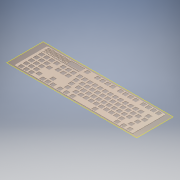
# Autodesk Inventor part: Plate
Saved by Autodesk Inventor 2016 (Build 200138000, 138)
## iProperties
Created: 2021-02-01
Part Number: Plate
Material: Aluminum 6061
Document SubType Name: Modeling
Designer: Tom
Density: 2.7 g/cm^3
Appearance: Aluminum - Flat
Author: Tom
Autodesk Inventor part; units mm, degrees
(part 1 of 4)
ref_plane "YZ Plane" through (0, 0, 0) normal (1, 0, 0) x (0, 1, 0)
ref_plane "XZ Plane" through (0, 0, 0) normal (0, 1, 0) x (-1, 0, 0)
ref_plane "XY Plane" through (0, 0, 0) normal (0, 0, 1) x (1, 0, 0)
ref_plane "Work Plane1" through (-107.46, -92.5006, 10.9251) normal (0, 0, 1) x (1, 0, 0)
sketch "Sketch1" plane through (-107.46, -92.5006, 10.9251) normal (0, 0, 1) x (1, 0, 0)
  line L0 (216.125, 61.75) -> (-216.125, 61.75)
  arc A0 (-216.125, 61.75) -> (-220.875, 57) centre (-216.125, 57) ccw
  line L1 (-220.875, 57) -> (-220.875, -57)
  arc A1 (-220.875, -57) -> (-216.125, -61.75) centre (-216.125, -57) ccw
  line L2 (-216.125, -61.75) -> (216.125, -61.75)
  arc A2 (216.125, -61.75) -> (220.875, -57) centre (216.125, -57) ccw
  line L3 (220.875, -57) -> (220.875, 57)
  arc A3 (220.875, 57) -> (216.125, 61.75) centre (216.125, 57) ccw
  circle A4 centre (216.125, 57) radius 1.35
  circle A5 centre (216.125, 0) radius 1.35
  circle A6 centre (216.125, -57) radius 1.35
  circle A7 centre (118.75, -57) radius 1.35
  circle A8 centre (23.75, -57) radius 1.35
  circle A9 centre (-133.753, -57) radius 1.35
  circle A10 centre (-47.5, -57) radius 1.35
  circle A11 centre (-216.125, -57) radius 1.35
  circle A12 centre (-216.125, 57) radius 1.35
  circle A13 centre (-216.125, 0) radius 1.35
  circle A14 centre (-66.5, -19) radius 1.35
  circle A15 centre (-45.125, 11.875) radius 1.35
  circle A16 centre (-73.625, 57) radius 1.35
  circle A17 centre (-9.5, -24.356) radius 1.35
  circle A18 centre (47.5, 57) radius 1.35
  circle A19 centre (-114, 14.25) radius 1.35
  circle A20 centre (-175.75, 14.25) radius 1.35
  circle A21 centre (-175.75, -23.75) radius 1.35
  circle A22 centre (33.25, 13.49) radius 1.35
  circle A23 centre (76, -23.086) radius 1.35
  circle A24 centre (109.25, 13.49) radius 1.35
  circle A25 centre (166.25, -40.375) radius 1.35
  circle A26 centre (187.625, 11.875) radius 1.35
  circle A27 centre (133, 57) radius 1.35
  line L4 (-78.04, 59.315) -> (-128.84, 59.315)
  line L5 (-128.84, 41.535) -> (-78.04, 41.535)
  line L6 (-78.04, 56.315) -> (-78.04, 44.535)
  line L7 (-78.04, 56.315) -> (-78.04, 59.315)
  line L8 (-78.04, 41.535) -> (-78.04, 44.535)
  line L9 (-128.84, 44.535) -> (-128.84, 41.535)
  line L10 (-128.84, 59.315) -> (-128.84, 56.315)
  line L11 (-128.84, 56.315) -> (-128.84, 44.535)
  line L12 (-78.04, 59.315) -> (-77.34, 59.315)
  line L13 (-77.34, 59.315) -> (-77.34, 41.535)
  line L14 (-77.34, 41.535) -> (-78.04, 41.535)
  line L15 (-128.84, 59.315) -> (-129.54, 59.315)
  line L16 (-129.54, 59.315) -> (-129.54, 41.535)
  line L17 (-129.54, 41.535) -> (-128.84, 41.535)
  line L18 (-62.2, 51.5) -> (-62.2, 50.35)
  line L19 (-62.2, 50.35) -> (-61.3, 50.35)
  line L20 (-61.3, 50.35) -> (-61.3, 51.5)
  arc A28 (-61.1, 51.7) -> (-61.3, 51.5) centre (-61.1, 51.5) ccw
  line L21 (-61.1, 51.7) -> (-59.85, 51.7)
  line L22 (-59.85, 51.7) -> (-59.85, 52.8)
  line L23 (-59.85, 52.8) -> (-61.1, 52.8)
  arc A29 (-61.3, 53) -> (-61.1, 52.8) centre (-61.1, 53) ccw
  line L24 (-61.3, 53) -> (-61.3, 54.15)
  line L25 (-61.3, 54.15) -> (-62.2, 54.15)
  line L26 (-62.2, 54.15) -> (-62.2, 53)
  arc A30 (-62.4, 52.8) -> (-62.2, 53) centre (-62.4, 53) ccw
  line L27 (-62.4, 52.8) -> (-63.65, 52.8)
  line L28 (-63.65, 52.8) -> (-63.65, 51.7)
  line L29 (-63.65, 51.7) -> (-62.4, 51.7)
  arc A31 (-62.2, 51.5) -> (-62.4, 51.7) centre (-62.4, 51.5) ccw
  line L30 (-24.2, 51.5) -> (-24.2, 50.35)
  line L31 (-24.2, 50.35) -> (-23.3, 50.35)
  line L32 (-23.3, 50.35) -> (-23.3, 51.5)
  arc A32 (-23.1, 51.7) -> (-23.3, 51.5) centre (-23.1, 51.5) ccw
  line L33 (-23.1, 51.7) -> (-21.85, 51.7)
  line L34 (-21.85, 51.7) -> (-21.85, 52.8)
  line L35 (-21.85, 52.8) -> (-23.1, 52.8)
  arc A33 (-23.3, 53) -> (-23.1, 52.8) centre (-23.1, 53) ccw
  line L36 (-23.3, 53) -> (-23.3, 54.15)
  line L37 (-23.3, 54.15) -> (-24.2, 54.15)
  line L38 (-24.2, 54.15) -> (-24.2, 53)
  arc A34 (-24.4, 52.8) -> (-24.2, 53) centre (-24.4, 53) ccw
  line L39 (-24.4, 52.8) -> (-25.65, 52.8)
  line L40 (-25.65, 52.8) -> (-25.65, 51.7)
  line L41 (-25.65, 51.7) -> (-24.4, 51.7)
  arc A35 (-24.2, 51.5) -> (-24.4, 51.7) centre (-24.4, 51.5) ccw
  line L42 (-24.2, 23) -> (-24.2, 21.85)
  line L43 (-24.2, 21.85) -> (-23.3, 21.85)
  line L44 (-23.3, 21.85) -> (-23.3, 23)
  arc A36 (-23.1, 23.2) -> (-23.3, 23) centre (-23.1, 23) ccw
  line L45 (-23.1, 23.2) -> (-21.85, 23.2)
  line L46 (-21.85, 23.2) -> (-21.85, 24.3)
  line L47 (-21.85, 24.3) -> (-23.1, 24.3)
  arc A37 (-23.3, 24.5) -> (-23.1, 24.3) centre (-23.1, 24.5) ccw
  line L48 (-23.3, 24.5) -> (-23.3, 25.65)
  line L49 (-23.3, 25.65) -> (-24.2, 25.65)
  line L50 (-24.2, 25.65) -> (-24.2, 24.5)
  arc A38 (-24.4, 24.3) -> (-24.2, 24.5) centre (-24.4, 24.5) ccw
  line L51 (-24.4, 24.3) -> (-25.65, 24.3)
  line L52 (-25.65, 24.3) -> (-25.65, 23.2)
  line L53 (-25.65, 23.2) -> (-24.4, 23.2)
  arc A39 (-24.2, 23) -> (-24.4, 23.2) centre (-24.4, 23) ccw
  line L54 (-43.2, 23) -> (-43.2, 21.85)
  line L55 (-43.2, 21.85) -> (-42.3, 21.85)
  line L56 (-42.3, 21.85) -> (-42.3, 23)
  arc A40 (-42.1, 23.2) -> (-42.3, 23) centre (-42.1, 23) ccw
  line L57 (-42.1, 23.2) -> (-40.85, 23.2)
  line L58 (-40.85, 23.2) -> (-40.85, 24.3)
  line L59 (-40.85, 24.3) -> (-42.1, 24.3)
  arc A41 (-42.3, 24.5) -> (-42.1, 24.3) centre (-42.1, 24.5) ccw
  line L60 (-42.3, 24.5) -> (-42.3, 25.65)
  line L61 (-42.3, 25.65) -> (-43.2, 25.65)
  line L62 (-43.2, 25.65) -> (-43.2, 24.5)
  arc A42 (-43.4, 24.3) -> (-43.2, 24.5) centre (-43.4, 24.5) ccw
  line L63 (-43.4, 24.3) -> (-44.65, 24.3)
  line L64 (-44.65, 24.3) -> (-44.65, 23.2)
  line L65 (-44.65, 23.2) -> (-43.4, 23.2)
  arc A43 (-43.2, 23) -> (-43.4, 23.2) centre (-43.4, 23) ccw
  line L66 (-62.2, 23) -> (-62.2, 21.85)
  line L67 (-62.2, 21.85) -> (-61.3, 21.85)
  line L68 (-61.3, 21.85) -> (-61.3, 23)
  arc A44 (-61.1, 23.2) -> (-61.3, 23) centre (-61.1, 23) ccw
  line L69 (-61.1, 23.2) -> (-59.85, 23.2)
  line L70 (-59.85, 23.2) -> (-59.85, 24.3)
  line L71 (-59.85, 24.3) -> (-61.1, 24.3)
  arc A45 (-61.3, 24.5) -> (-61.1, 24.3) centre (-61.1, 24.5) ccw
  line L72 (-61.3, 24.5) -> (-61.3, 25.65)
  line L73 (-61.3, 25.65) -> (-62.2, 25.65)
  line L74 (-62.2, 25.65) -> (-62.2, 24.5)
  arc A46 (-62.4, 24.3) -> (-62.2, 24.5) centre (-62.4, 24.5) ccw
  line L75 (-62.4, 24.3) -> (-63.65, 24.3)
  line L76 (-63.65, 24.3) -> (-63.65, 23.2)
  line L77 (-63.65, 23.2) -> (-62.4, 23.2)
  arc A47 (-62.2, 23) -> (-62.4, 23.2) centre (-62.4, 23) ccw
  line L78 (-123.95, 23) -> (-123.95, 21.85)
  line L79 (-123.95, 21.85) -> (-123.05, 21.85)
  line L80 (-123.05, 21.85) -> (-123.05, 23)
  arc A48 (-122.85, 23.2) -> (-123.05, 23) centre (-122.85, 23) ccw
  line L81 (-122.85, 23.2) -> (-121.6, 23.2)
  line L82 (-121.6, 23.2) -> (-121.6, 24.3)
  line L83 (-121.6, 24.3) -> (-122.85, 24.3)
  arc A49 (-123.05, 24.5) -> (-122.85, 24.3) centre (-122.85, 24.5) ccw
  line L84 (-123.05, 24.5) -> (-123.05, 25.65)
  line L85 (-123.05, 25.65) -> (-123.95, 25.65)
  line L86 (-123.95, 25.65) -> (-123.95, 24.5)
  arc A50 (-124.15, 24.3) -> (-123.95, 24.5) centre (-124.15, 24.5) ccw
  line L87 (-124.15, 24.3) -> (-125.4, 24.3)
  line L88 (-125.4, 24.3) -> (-125.4, 23.2)
  line L89 (-125.4, 23.2) -> (-124.15, 23.2)
  arc A51 (-123.95, 23) -> (-124.15, 23.2) centre (-124.15, 23) ccw
  line L90 (-104.95, 23) -> (-104.95, 21.85)
  line L91 (-104.95, 21.85) -> (-104.05, 21.85)
  line L92 (-104.05, 21.85) -> (-104.05, 23)
  arc A52 (-103.85, 23.2) -> (-104.05, 23) centre (-103.85, 23) ccw
  line L93 (-103.85, 23.2) -> (-102.6, 23.2)
  line L94 (-102.6, 23.2) -> (-102.6, 24.3)
  line L95 (-102.6, 24.3) -> (-103.85, 24.3)
  arc A53 (-104.05, 24.5) -> (-103.85, 24.3) centre (-103.85, 24.5) ccw
  line L96 (-104.05, 24.5) -> (-104.05, 25.65)
  line L97 (-104.05, 25.65) -> (-104.95, 25.65)
  line L98 (-104.95, 25.65) -> (-104.95, 24.5)
  arc A54 (-105.15, 24.3) -> (-104.95, 24.5) centre (-105.15, 24.5) ccw
  line L99 (-105.15, 24.3) -> (-106.4, 24.3)
  line L100 (-106.4, 24.3) -> (-106.4, 23.2)
  line L101 (-106.4, 23.2) -> (-105.15, 23.2)
  arc A55 (-104.95, 23) -> (-105.15, 23.2) centre (-105.15, 23) ccw
  line L102 (-85.95, 23) -> (-85.95, 21.85)
  line L103 (-85.95, 21.85) -> (-85.05, 21.85)
  line L104 (-85.05, 21.85) -> (-85.05, 23)
  arc A56 (-84.85, 23.2) -> (-85.05, 23) centre (-84.85, 23) ccw
  line L105 (-84.85, 23.2) -> (-83.6, 23.2)
  line L106 (-83.6, 23.2) -> (-83.6, 24.3)
  line L107 (-83.6, 24.3) -> (-84.85, 24.3)
  arc A57 (-85.05, 24.5) -> (-84.85, 24.3) centre (-84.85, 24.5) ccw
  line L108 (-85.05, 24.5) -> (-85.05, 25.65)
  line L109 (-85.05, 25.65) -> (-85.95, 25.65)
  line L110 (-85.95, 25.65) -> (-85.95, 24.5)
  arc A58 (-86.15, 24.3) -> (-85.95, 24.5) centre (-86.15, 24.5) ccw
  line L111 (-86.15, 24.3) -> (-87.4, 24.3)
  line L112 (-87.4, 24.3) -> (-87.4, 23.2)
  line L113 (-87.4, 23.2) -> (-86.15, 23.2)
  arc A59 (-85.95, 23) -> (-86.15, 23.2) centre (-86.15, 23) ccw
  line L114 (-85.95, 4) -> (-85.95, 2.85)
  line L115 (-85.95, 2.85) -> (-85.05, 2.85)
  line L116 (-85.05, 2.85) -> (-85.05, 4)
  arc A60 (-84.85, 4.2) -> (-85.05, 4) centre (-84.85, 4) ccw
  line L117 (-84.85, 4.2) -> (-83.6, 4.2)
  line L118 (-83.6, 4.2) -> (-83.6, 5.3)
  line L119 (-83.6, 5.3) -> (-84.85, 5.3)
  arc A61 (-85.05, 5.5) -> (-84.85, 5.3) centre (-84.85, 5.5) ccw
  line L120 (-85.05, 5.5) -> (-85.05, 6.65)
  line L121 (-85.05, 6.65) -> (-85.95, 6.65)
  line L122 (-85.95, 6.65) -> (-85.95, 5.5)
  arc A62 (-86.15, 5.3) -> (-85.95, 5.5) centre (-86.15, 5.5) ccw
  line L123 (-86.15, 5.3) -> (-87.4, 5.3)
  line L124 (-87.4, 5.3) -> (-87.4, 4.2)
  line L125 (-87.4, 4.2) -> (-86.15, 4.2)
  arc A63 (-85.95, 4) -> (-86.15, 4.2) centre (-86.15, 4) ccw
  line L126 (-104.95, 4) -> (-104.95, 2.85)
  line L127 (-104.95, 2.85) -> (-104.05, 2.85)
  line L128 (-104.05, 2.85) -> (-104.05, 4)
  arc A64 (-103.85, 4.2) -> (-104.05, 4) centre (-103.85, 4) ccw
  line L129 (-103.85, 4.2) -> (-102.6, 4.2)
  line L130 (-102.6, 4.2) -> (-102.6, 5.3)
  line L131 (-102.6, 5.3) -> (-103.85, 5.3)
  arc A65 (-104.05, 5.5) -> (-103.85, 5.3) centre (-103.85, 5.5) ccw
  line L132 (-104.05, 5.5) -> (-104.05, 6.65)
  line L133 (-104.05, 6.65) -> (-104.95, 6.65)
  line L134 (-104.95, 6.65) -> (-104.95, 5.5)
  arc A66 (-105.15, 5.3) -> (-104.95, 5.5) centre (-105.15, 5.5) ccw
  line L135 (-105.15, 5.3) -> (-106.4, 5.3)
  line L136 (-106.4, 5.3) -> (-106.4, 4.2)
  line L137 (-106.4, 4.2) -> (-105.15, 4.2)
  arc A67 (-104.95, 4) -> (-105.15, 4.2) centre (-105.15, 4) ccw
  line L138 (-123.95, 4) -> (-123.95, 2.85)
  line L139 (-123.95, 2.85) -> (-123.05, 2.85)
  line L140 (-123.05, 2.85) -> (-123.05, 4)
  arc A68 (-122.85, 4.2) -> (-123.05, 4) centre (-122.85, 4) ccw
  line L141 (-122.85, 4.2) -> (-121.6, 4.2)
  line L142 (-121.6, 4.2) -> (-121.6, 5.3)
  line L143 (-121.6, 5.3) -> (-122.85, 5.3)
  arc A69 (-123.05, 5.5) -> (-122.85, 5.3) centre (-122.85, 5.5) ccw
  line L144 (-123.05, 5.5) -> (-123.05, 6.65)
  line L145 (-123.05, 6.65) -> (-123.95, 6.65)
  line L146 (-123.95, 6.65) -> (-123.95, 5.5)
  arc A70 (-124.15, 5.3) -> (-123.95, 5.5) centre (-124.15, 5.5) ccw
  line L147 (-124.15, 5.3) -> (-125.4, 5.3)
  line L148 (-125.4, 5.3) -> (-125.4, 4.2)
  line L149 (-125.4, 4.2) -> (-124.15, 4.2)
  arc A71 (-123.95, 4) -> (-124.15, 4.2) centre (-124.15, 4) ccw
  line L150 (32.8, 51.5) -> (32.8, 50.35)
  line L151 (32.8, 50.35) -> (33.7, 50.35)
  line L152 (33.7, 50.35) -> (33.7, 51.5)
  arc A72 (33.9, 51.7) -> (33.7, 51.5) centre (33.9, 51.5) ccw
  line L153 (33.9, 51.7) -> (35.15, 51.7)
  line L154 (35.15, 51.7) -> (35.15, 52.8)
  line L155 (35.15, 52.8) -> (33.9, 52.8)
  arc A73 (33.7, 53) -> (33.9, 52.8) centre (33.9, 53) ccw
  line L156 (33.7, 53) -> (33.7, 54.15)
  line L157 (33.7, 54.15) -> (32.8, 54.15)
  line L158 (32.8, 54.15) -> (32.8, 53)
  arc A74 (32.6, 52.8) -> (32.8, 53) centre (32.6, 53) ccw
  line L159 (32.6, 52.8) -> (31.35, 52.8)
  line L160 (31.35, 52.8) -> (31.35, 51.7)
  line L161 (31.35, 51.7) -> (32.6, 51.7)
  arc A75 (32.8, 51.5) -> (32.6, 51.7) centre (32.6, 51.5) ccw
  line L162 (13.8, 51.5) -> (13.8, 50.35)
  line L163 (13.8, 50.35) -> (14.7, 50.35)
  line L164 (14.7, 50.35) -> (14.7, 51.5)
  arc A76 (14.9, 51.7) -> (14.7, 51.5) centre (14.9, 51.5) ccw
  line L165 (14.9, 51.7) -> (16.15, 51.7)
  line L166 (16.15, 51.7) -> (16.15, 52.8)
  line L167 (16.15, 52.8) -> (14.9, 52.8)
  arc A77 (14.7, 53) -> (14.9, 52.8) centre (14.9, 53) ccw
  line L168 (14.7, 53) -> (14.7, 54.15)
  line L169 (14.7, 54.15) -> (13.8, 54.15)
  line L170 (13.8, 54.15) -> (13.8, 53)
  arc A78 (13.6, 52.8) -> (13.8, 53) centre (13.6, 53) ccw
  line L171 (13.6, 52.8) -> (12.35, 52.8)
  line L172 (12.35, 52.8) -> (12.35, 51.7)
  line L173 (12.35, 51.7) -> (13.6, 51.7)
  arc A79 (13.8, 51.5) -> (13.6, 51.7) centre (13.6, 51.5) ccw
  line L174 (-5.2, 51.5) -> (-5.2, 50.35)
  line L175 (-5.2, 50.35) -> (-4.3, 50.35)
  line L176 (-4.3, 50.35) -> (-4.3, 51.5)
  arc A80 (-4.1, 51.7) -> (-4.3, 51.5) centre (-4.1, 51.5) ccw
  line L177 (-4.1, 51.7) -> (-2.85, 51.7)
  line L178 (-2.85, 51.7) -> (-2.85, 52.8)
  line L179 (-2.85, 52.8) -> (-4.1, 52.8)
  arc A81 (-4.3, 53) -> (-4.1, 52.8) centre (-4.1, 53) ccw
  line L180 (-4.3, 53) -> (-4.3, 54.15)
  line L181 (-4.3, 54.15) -> (-5.2, 54.15)
  line L182 (-5.2, 54.15) -> (-5.2, 53)
  arc A82 (-5.4, 52.8) -> (-5.2, 53) centre (-5.4, 53) ccw
  line L183 (-5.4, 52.8) -> (-6.65, 52.8)
  line L184 (-6.65, 52.8) -> (-6.65, 51.7)
  line L185 (-6.65, 51.7) -> (-5.4, 51.7)
  arc A83 (-5.2, 51.5) -> (-5.4, 51.7) centre (-5.4, 51.5) ccw
  line L186 (-5.2, 23) -> (-5.2, 21.85)
  line L187 (-5.2, 21.85) -> (-4.3, 21.85)
  line L188 (-4.3, 21.85) -> (-4.3, 23)
  arc A84 (-4.1, 23.2) -> (-4.3, 23) centre (-4.1, 23) ccw
  line L189 (-4.1, 23.2) -> (-2.85, 23.2)
  line L190 (-2.85, 23.2) -> (-2.85, 24.3)
  line L191 (-2.85, 24.3) -> (-4.1, 24.3)
  arc A85 (-4.3, 24.5) -> (-4.1, 24.3) centre (-4.1, 24.5) ccw
  line L192 (-4.3, 24.5) -> (-4.3, 25.65)
  line L193 (-4.3, 25.65) -> (-5.2, 25.65)
  line L194 (-5.2, 25.65) -> (-5.2, 24.5)
  arc A86 (-5.4, 24.3) -> (-5.2, 24.5) centre (-5.4, 24.5) ccw
  line L195 (-5.4, 24.3) -> (-6.65, 24.3)
  line L196 (-6.65, 24.3) -> (-6.65, 23.2)
  line L197 (-6.65, 23.2) -> (-5.4, 23.2)
  arc A87 (-5.2, 23) -> (-5.4, 23.2) centre (-5.4, 23) ccw
  line L198 (13.8, 23) -> (13.8, 21.85)
  line L199 (13.8, 21.85) -> (14.7, 21.85)
  line L200 (14.7, 21.85) -> (14.7, 23)
  arc A88 (14.9, 23.2) -> (14.7, 23) centre (14.9, 23) ccw
  line L201 (14.9, 23.2) -> (16.15, 23.2)
  line L202 (16.15, 23.2) -> (16.15, 24.3)
  line L203 (16.15, 24.3) -> (14.9, 24.3)
  arc A89 (14.7, 24.5) -> (14.9, 24.3) centre (14.9, 24.5) ccw
  line L204 (14.7, 24.5) -> (14.7, 25.65)
  line L205 (14.7, 25.65) -> (13.8, 25.65)
  line L206 (13.8, 25.65) -> (13.8, 24.5)
  arc A90 (13.6, 24.3) -> (13.8, 24.5) centre (13.6, 24.5) ccw
  line L207 (13.6, 24.3) -> (12.35, 24.3)
  line L208 (12.35, 24.3) -> (12.35, 23.2)
  line L209 (12.35, 23.2) -> (13.6, 23.2)
  arc A91 (13.8, 23) -> (13.6, 23.2) centre (13.6, 23) ccw
  line L210 (32.8, 23) -> (32.8, 21.85)
  line L211 (32.8, 21.85) -> (33.7, 21.85)
  line L212 (33.7, 21.85) -> (33.7, 23)
  arc A92 (33.9, 23.2) -> (33.7, 23) centre (33.9, 23) ccw
  line L213 (33.9, 23.2) -> (35.15, 23.2)
  line L214 (35.15, 23.2) -> (35.15, 24.3)
  line L215 (35.15, 24.3) -> (33.9, 24.3)
  arc A93 (33.7, 24.5) -> (33.9, 24.3) centre (33.9, 24.5) ccw
  line L216 (33.7, 24.5) -> (33.7, 25.65)
  line L217 (33.7, 25.65) -> (32.8, 25.65)
  line L218 (32.8, 25.65) -> (32.8, 24.5)
  arc A94 (32.6, 24.3) -> (32.8, 24.5) centre (32.6, 24.5) ccw
  line L219 (32.6, 24.3) -> (31.35, 24.3)
  line L220 (31.35, 24.3) -> (31.35, 23.2)
  line L221 (31.35, 23.2) -> (32.6, 23.2)
  arc A95 (32.8, 23) -> (32.6, 23.2) centre (32.6, 23) ccw
  line L222 (61.3, 51.5) -> (61.3, 50.35)
  line L223 (61.3, 50.35) -> (62.2, 50.35)
  line L224 (62.2, 50.35) -> (62.2, 51.5)
  arc A96 (62.4, 51.7) -> (62.2, 51.5) centre (62.4, 51.5) ccw
  line L225 (62.4, 51.7) -> (63.65, 51.7)
  line L226 (63.65, 51.7) -> (63.65, 52.8)
  line L227 (63.65, 52.8) -> (62.4, 52.8)
  arc A97 (62.2, 53) -> (62.4, 52.8) centre (62.4, 53) ccw
  line L228 (62.2, 53) -> (62.2, 54.15)
  line L229 (62.2, 54.15) -> (61.3, 54.15)
  line L230 (61.3, 54.15) -> (61.3, 53)
  arc A98 (61.1, 52.8) -> (61.3, 53) centre (61.1, 53) ccw
  line L231 (61.1, 52.8) -> (59.85, 52.8)
  line L232 (59.85, 52.8) -> (59.85, 51.7)
  line L233 (59.85, 51.7) -> (61.1, 51.7)
  arc A99 (61.3, 51.5) -> (61.1, 51.7) centre (61.1, 51.5) ccw
  line L234 (80.3, 51.5) -> (80.3, 50.35)
  line L235 (80.3, 50.35) -> (81.2, 50.35)
  line L236 (81.2, 50.35) -> (81.2, 51.5)
  arc A100 (81.4, 51.7) -> (81.2, 51.5) centre (81.4, 51.5) ccw
  line L237 (81.4, 51.7) -> (82.65, 51.7)
  line L238 (82.65, 51.7) -> (82.65, 52.8)
  line L239 (82.65, 52.8) -> (81.4, 52.8)
  arc A101 (81.2, 53) -> (81.4, 52.8) centre (81.4, 53) ccw
  line L240 (81.2, 53) -> (81.2, 54.15)
  line L241 (81.2, 54.15) -> (80.3, 54.15)
  line L242 (80.3, 54.15) -> (80.3, 53)
  arc A102 (80.1, 52.8) -> (80.3, 53) centre (80.1, 53) ccw
  line L243 (80.1, 52.8) -> (78.85, 52.8)
  line L244 (78.85, 52.8) -> (78.85, 51.7)
  line L245 (78.85, 51.7) -> (80.1, 51.7)
  arc A103 (80.3, 51.5) -> (80.1, 51.7) centre (80.1, 51.5) ccw
  line L246 (99.3, 51.5) -> (99.3, 50.35)
  line L247 (99.3, 50.35) -> (100.2, 50.35)
  line L248 (100.2, 50.35) -> (100.2, 51.5)
  arc A104 (100.4, 51.7) -> (100.2, 51.5) centre (100.4, 51.5) ccw
  line L249 (100.4, 51.7) -> (101.65, 51.7)
  line L250 (101.65, 51.7) -> (101.65, 52.8)
  line L251 (101.65, 52.8) -> (100.4, 52.8)
  arc A105 (100.2, 53) -> (100.4, 52.8) centre (100.4, 53) ccw
  line L252 (100.2, 53) -> (100.2, 54.15)
  line L253 (100.2, 54.15) -> (99.3, 54.15)
  line L254 (99.3, 54.15) -> (99.3, 53)
  arc A106 (99.1, 52.8) -> (99.3, 53) centre (99.1, 53) ccw
  line L255 (99.1, 52.8) -> (97.85, 52.8)
  line L256 (97.85, 52.8) -> (97.85, 51.7)
  line L257 (97.85, 51.7) -> (99.1, 51.7)
  arc A107 (99.3, 51.5) -> (99.1, 51.7) centre (99.1, 51.5) ccw
  line L258 (118.3, 51.5) -> (118.3, 50.35)
  line L259 (118.3, 50.35) -> (119.2, 50.35)
  line L260 (119.2, 50.35) -> (119.2, 51.5)
  arc A108 (119.4, 51.7) -> (119.2, 51.5) centre (119.4, 51.5) ccw
  line L261 (119.4, 51.7) -> (120.65, 51.7)
  line L262 (120.65, 51.7) -> (120.65, 52.8)
  line L263 (120.65, 52.8) -> (119.4, 52.8)
  arc A109 (119.2, 53) -> (119.4, 52.8) centre (119.4, 53) ccw
  line L264 (119.2, 53) -> (119.2, 54.15)
  line L265 (119.2, 54.15) -> (118.3, 54.15)
  line L266 (118.3, 54.15) -> (118.3, 53)
  arc A110 (118.1, 52.8) -> (118.3, 53) centre (118.1, 53) ccw
  line L267 (118.1, 52.8) -> (116.85, 52.8)
  line L268 (116.85, 52.8) -> (116.85, 51.7)
  line L269 (116.85, 51.7) -> (118.1, 51.7)
  arc A111 (118.3, 51.5) -> (118.1, 51.7) centre (118.1, 51.5) ccw
  line L270 (51.8, 23) -> (51.8, 21.85)
  line L271 (51.8, 21.85) -> (52.7, 21.85)
  line L272 (52.7, 21.85) -> (52.7, 23)
  arc A112 (52.9, 23.2) -> (52.7, 23) centre (52.9, 23) ccw
  line L273 (52.9, 23.2) -> (54.15, 23.2)
  line L274 (54.15, 23.2) -> (54.15, 24.3)
  line L275 (54.15, 24.3) -> (52.9, 24.3)
  arc A113 (52.7, 24.5) -> (52.9, 24.3) centre (52.9, 24.5) ccw
  line L276 (52.7, 24.5) -> (52.7, 25.65)
  line L277 (52.7, 25.65) -> (51.8, 25.65)
  line L278 (51.8, 25.65) -> (51.8, 24.5)
  arc A114 (51.6, 24.3) -> (51.8, 24.5) centre (51.6, 24.5) ccw
  line L279 (51.6, 24.3) -> (50.35, 24.3)
  line L280 (50.35, 24.3) -> (50.35, 23.2)
  line L281 (50.35, 23.2) -> (51.6, 23.2)
  arc A115 (51.8, 23) -> (51.6, 23.2) centre (51.6, 23) ccw
  line L282 (70.8, 23) -> (70.8, 21.85)
  line L283 (70.8, 21.85) -> (71.7, 21.85)
  line L284 (71.7, 21.85) -> (71.7, 23)
  arc A116 (71.9, 23.2) -> (71.7, 23) centre (71.9, 23) ccw
  line L285 (71.9, 23.2) -> (73.15, 23.2)
  line L286 (73.15, 23.2) -> (73.15, 24.3)
  line L287 (73.15, 24.3) -> (71.9, 24.3)
  arc A117 (71.7, 24.5) -> (71.9, 24.3) centre (71.9, 24.5) ccw
  line L288 (71.7, 24.5) -> (71.7, 25.65)
  line L289 (71.7, 25.65) -> (70.8, 25.65)
  line L290 (70.8, 25.65) -> (70.8, 24.5)
  arc A118 (70.6, 24.3) -> (70.8, 24.5) centre (70.6, 24.5) ccw
  line L291 (70.6, 24.3) -> (69.35, 24.3)
  line L292 (69.35, 24.3) -> (69.35, 23.2)
  line L293 (69.35, 23.2) -> (70.6, 23.2)
  arc A119 (70.8, 23) -> (70.6, 23.2) centre (70.6, 23) ccw
  line L294 (89.8, 23) -> (89.8, 21.85)
  line L295 (89.8, 21.85) -> (90.7, 21.85)
  line L296 (90.7, 21.85) -> (90.7, 23)
  arc A120 (90.9, 23.2) -> (90.7, 23) centre (90.9, 23) ccw
  line L297 (90.9, 23.2) -> (92.15, 23.2)
  line L298 (92.15, 23.2) -> (92.15, 24.3)
  line L299 (92.15, 24.3) -> (90.9, 24.3)
  arc A121 (90.7, 24.5) -> (90.9, 24.3) centre (90.9, 24.5) ccw
  line L300 (90.7, 24.5) -> (90.7, 25.65)
  line L301 (90.7, 25.65) -> (89.8, 25.65)
  line L302 (89.8, 25.65) -> (89.8, 24.5)
  arc A122 (89.6, 24.3) -> (89.8, 24.5) centre (89.6, 24.5) ccw
  line L303 (89.6, 24.3) -> (88.35, 24.3)
  line L304 (88.35, 24.3) -> (88.35, 23.2)
  line L305 (88.35, 23.2) -> (89.6, 23.2)
  arc A123 (89.8, 23) -> (89.6, 23.2) centre (89.6, 23) ccw
  line L306 (108.8, 23) -> (108.8, 21.85)
  line L307 (108.8, 21.85) -> (109.7, 21.85)
  line L308 (109.7, 21.85) -> (109.7, 23)
  arc A124 (109.9, 23.2) -> (109.7, 23) centre (109.9, 23) ccw
  line L309 (109.9, 23.2) -> (111.15, 23.2)
  line L310 (111.15, 23.2) -> (111.15, 24.3)
  line L311 (111.15, 24.3) -> (109.9, 24.3)
  arc A125 (109.7, 24.5) -> (109.9, 24.3) centre (109.9, 24.5) ccw
  line L312 (109.7, 24.5) -> (109.7, 25.65)
  line L313 (109.7, 25.65) -> (108.8, 25.65)
  line L314 (108.8, 25.65) -> (108.8, 24.5)
  arc A126 (108.6, 24.3) -> (108.8, 24.5) centre (108.6, 24.5) ccw
  line L315 (108.6, 24.3) -> (107.35, 24.3)
  line L316 (107.35, 24.3) -> (107.35, 23.2)
  line L317 (107.35, 23.2) -> (108.6, 23.2)
  arc A127 (108.8, 23) -> (108.6, 23.2) centre (108.6, 23) ccw
  line L318 (127.8, 23) -> (127.8, 21.85)
  line L319 (127.8, 21.85) -> (128.7, 21.85)
  line L320 (128.7, 21.85) -> (128.7, 23)
  arc A128 (128.9, 23.2) -> (128.7, 23) centre (128.9, 23) ccw
  line L321 (128.9, 23.2) -> (130.15, 23.2)
  line L322 (130.15, 23.2) -> (130.15, 24.3)
  line L323 (130.15, 24.3) -> (128.9, 24.3)
  arc A129 (128.7, 24.5) -> (128.9, 24.3) centre (128.9, 24.5) ccw
  line L324 (128.7, 24.5) -> (128.7, 25.65)
  line L325 (128.7, 25.65) -> (127.8, 25.65)
  line L326 (127.8, 25.65) -> (127.8, 24.5)
  arc A130 (127.6, 24.3) -> (127.8, 24.5) centre (127.6, 24.5) ccw
  line L327 (127.6, 24.3) -> (126.35, 24.3)
  line L328 (126.35, 24.3) -> (126.35, 23.2)
  line L329 (126.35, 23.2) -> (127.6, 23.2)
  arc A131 (127.8, 23) -> (127.6, 23.2) centre (127.6, 23) ccw
  line L330 (146.8, 23) -> (146.8, 21.85)
  line L331 (146.8, 21.85) -> (147.7, 21.85)
  line L332 (147.7, 21.85) -> (147.7, 23)
  arc A132 (147.9, 23.2) -> (147.7, 23) centre (147.9, 23) ccw
  line L333 (147.9, 23.2) -> (149.15, 23.2)
  line L334 (149.15, 23.2) -> (149.15, 24.3)
  line L335 (149.15, 24.3) -> (147.9, 24.3)
  arc A133 (147.7, 24.5) -> (147.9, 24.3) centre (147.9, 24.5) ccw
  line L336 (147.7, 24.5) -> (147.7, 25.65)
  line L337 (147.7, 25.65) -> (146.8, 25.65)
  line L338 (146.8, 25.65) -> (146.8, 24.5)
  arc A134 (146.6, 24.3) -> (146.8, 24.5) centre (146.6, 24.5) ccw
  line L339 (146.6, 24.3) -> (145.35, 24.3)
  line L340 (145.35, 24.3) -> (145.35, 23.2)
  line L341 (145.35, 23.2) -> (146.6, 23.2)
  arc A135 (146.8, 23) -> (146.6, 23.2) centre (146.6, 23) ccw
  line L342 (146.8, 51.5) -> (146.8, 50.35)
  line L343 (146.8, 50.35) -> (147.7, 50.35)
  line L344 (147.7, 50.35) -> (147.7, 51.5)
  arc A136 (147.9, 51.7) -> (147.7, 51.5) centre (147.9, 51.5) ccw
  line L345 (147.9, 51.7) -> (149.15, 51.7)
  line L346 (149.15, 51.7) -> (149.15, 52.8)
  line L347 (149.15, 52.8) -> (147.9, 52.8)
  arc A137 (147.7, 53) -> (147.9, 52.8) centre (147.9, 53) ccw
  line L348 (147.7, 53) -> (147.7, 54.15)
  line L349 (147.7, 54.15) -> (146.8, 54.15)
  line L350 (146.8, 54.15) -> (146.8, 53)
  arc A138 (146.6, 52.8) -> (146.8, 53) centre (146.6, 53) ccw
  line L351 (146.6, 52.8) -> (145.35, 52.8)
  line L352 (145.35, 52.8) -> (145.35, 51.7)
  line L353 (145.35, 51.7) -> (146.6, 51.7)
  arc A139 (146.8, 51.5) -> (146.6, 51.7) centre (146.6, 51.5) ccw
  line L354 (165.8, 51.5) -> (165.8, 50.35)
  line L355 (165.8, 50.35) -> (166.7, 50.35)
  line L356 (166.7, 50.35) -> (166.7, 51.5)
  arc A140 (166.9, 51.7) -> (166.7, 51.5) centre (166.9, 51.5) ccw
  line L357 (166.9, 51.7) -> (168.15, 51.7)
  line L358 (168.15, 51.7) -> (168.15, 52.8)
  line L359 (168.15, 52.8) -> (166.9, 52.8)
  arc A141 (166.7, 53) -> (166.9, 52.8) centre (166.9, 53) ccw
  line L360 (166.7, 53) -> (166.7, 54.15)
  line L361 (166.7, 54.15) -> (165.8, 54.15)
  line L362 (165.8, 54.15) -> (165.8, 53)
  arc A142 (165.6, 52.8) -> (165.8, 53) centre (165.6, 53) ccw
  line L363 (165.6, 52.8) -> (164.35, 52.8)
  line L364 (164.35, 52.8) -> (164.35, 51.7)
  line L365 (164.35, 51.7) -> (165.6, 51.7)
  arc A143 (165.8, 51.5) -> (165.6, 51.7) centre (165.6, 51.5) ccw
  line L366 (184.8, 51.5) -> (184.8, 50.35)
  line L367 (184.8, 50.35) -> (185.7, 50.35)
  line L368 (185.7, 50.35) -> (185.7, 51.5)
  arc A144 (185.9, 51.7) -> (185.7, 51.5) centre (185.9, 51.5) ccw
  line L369 (185.9, 51.7) -> (187.15, 51.7)
  line L370 (187.15, 51.7) -> (187.15, 52.8)
  line L371 (187.15, 52.8) -> (185.9, 52.8)
  arc A145 (185.7, 53) -> (185.9, 52.8) centre (185.9, 53) ccw
  line L372 (185.7, 53) -> (185.7, 54.15)
  line L373 (185.7, 54.15) -> (184.8, 54.15)
  line L374 (184.8, 54.15) -> (184.8, 53)
  arc A146 (184.6, 52.8) -> (184.8, 53) centre (184.6, 53) ccw
  line L375 (184.6, 52.8) -> (183.35, 52.8)
  line L376 (183.35, 52.8) -> (183.35, 51.7)
  line L377 (183.35, 51.7) -> (184.6, 51.7)
  arc A147 (184.8, 51.5) -> (184.6, 51.7) centre (184.6, 51.5) ccw
  line L378 (203.8, 51.5) -> (203.8, 50.35)
  line L379 (203.8, 50.35) -> (204.7, 50.35)
  line L380 (204.7, 50.35) -> (204.7, 51.5)
  arc A148 (204.9, 51.7) -> (204.7, 51.5) centre (204.9, 51.5) ccw
  line L381 (204.9, 51.7) -> (206.15, 51.7)
  line L382 (206.15, 51.7) -> (206.15, 52.8)
  line L383 (206.15, 52.8) -> (204.9, 52.8)
  arc A149 (204.7, 53) -> (204.9, 52.8) centre (204.9, 53) ccw
  line L384 (204.7, 53) -> (204.7, 54.15)
  line L385 (204.7, 54.15) -> (203.8, 54.15)
  line L386 (203.8, 54.15) -> (203.8, 53)
  arc A150 (203.6, 52.8) -> (203.8, 53) centre (203.6, 53) ccw
  line L387 (203.6, 52.8) -> (202.35, 52.8)
  line L388 (202.35, 52.8) -> (202.35, 51.7)
  line L389 (202.35, 51.7) -> (203.6, 51.7)
  arc A151 (203.8, 51.5) -> (203.6, 51.7) centre (203.6, 51.5) ccw
  line L390 (194.3, 23) -> (194.3, 21.85)
  line L391 (194.3, 21.85) -> (195.2, 21.85)
  line L392 (195.2, 21.85) -> (195.2, 23)
  arc A152 (195.4, 23.2) -> (195.2, 23) centre (195.4, 23) ccw
  line L393 (195.4, 23.2) -> (196.65, 23.2)
  line L394 (196.65, 23.2) -> (196.65, 24.3)
  line L395 (196.65, 24.3) -> (195.4, 24.3)
  arc A153 (195.2, 24.5) -> (195.4, 24.3) centre (195.4, 24.5) ccw
  line L396 (195.2, 24.5) -> (195.2, 25.65)
  line L397 (195.2, 25.65) -> (194.3, 25.65)
  line L398 (194.3, 25.65) -> (194.3, 24.5)
  arc A154 (194.1, 24.3) -> (194.3, 24.5) centre (194.1, 24.5) ccw
  line L399 (194.1, 24.3) -> (192.85, 24.3)
  line L400 (192.85, 24.3) -> (192.85, 23.2)
  line L401 (192.85, 23.2) -> (194.1, 23.2)
  arc A155 (194.3, 23) -> (194.1, 23.2) centre (194.1, 23) ccw
  line L402 (165.8, 23) -> (165.8, 21.85)
  line L403 (165.8, 21.85) -> (166.7, 21.85)
  line L404 (166.7, 21.85) -> (166.7, 23)
  arc A156 (166.9, 23.2) -> (166.7, 23) centre (166.9, 23) ccw
  line L405 (166.9, 23.2) -> (168.15, 23.2)
  line L406 (168.15, 23.2) -> (168.15, 24.3)
  line L407 (168.15, 24.3) -> (166.9, 24.3)
  arc A157 (166.7, 24.5) -> (166.9, 24.3) centre (166.9, 24.5) ccw
  line L408 (166.7, 24.5) -> (166.7, 25.65)
  line L409 (166.7, 25.65) -> (165.8, 25.65)
  line L410 (165.8, 25.65) -> (165.8, 24.5)
  arc A158 (165.6, 24.3) -> (165.8, 24.5) centre (165.6, 24.5) ccw
  line L411 (165.6, 24.3) -> (164.35, 24.3)
  line L412 (164.35, 24.3) -> (164.35, 23.2)
  line L413 (164.35, 23.2) -> (165.6, 23.2)
  arc A159 (165.8, 23) -> (165.6, 23.2) centre (165.6, 23) ccw
  line L414 (-204.7, 23) -> (-204.7, 21.85)
  line L415 (-204.7, 21.85) -> (-203.8, 21.85)
  line L416 (-203.8, 21.85) -> (-203.8, 23)
  arc A160 (-203.6, 23.2) -> (-203.8, 23) centre (-203.6, 23) ccw
  line L417 (-203.6, 23.2) -> (-202.35, 23.2)
  line L418 (-202.35, 23.2) -> (-202.35, 24.3)
  line L419 (-202.35, 24.3) -> (-203.6, 24.3)
  arc A161 (-203.8, 24.5) -> (-203.6, 24.3) centre (-203.6, 24.5) ccw
  line L420 (-203.8, 24.5) -> (-203.8, 25.65)
  line L421 (-203.8, 25.65) -> (-204.7, 25.65)
  line L422 (-204.7, 25.65) -> (-204.7, 24.5)
  arc A162 (-204.9, 24.3) -> (-204.7, 24.5) centre (-204.9, 24.5) ccw
  line L423 (-204.9, 24.3) -> (-206.15, 24.3)
  line L424 (-206.15, 24.3) -> (-206.15, 23.2)
  line L425 (-206.15, 23.2) -> (-204.9, 23.2)
  arc A163 (-204.7, 23) -> (-204.9, 23.2) centre (-204.9, 23) ccw
  line L426 (-185.7, 23) -> (-185.7, 21.85)
  line L427 (-185.7, 21.85) -> (-184.8, 21.85)
  line L428 (-184.8, 21.85) -> (-184.8, 23)
  arc A164 (-184.6, 23.2) -> (-184.8, 23) centre (-184.6, 23) ccw
  line L429 (-184.6, 23.2) -> (-183.35, 23.2)
  line L430 (-183.35, 23.2) -> (-183.35, 24.3)
  line L431 (-183.35, 24.3) -> (-184.6, 24.3)
  arc A165 (-184.8, 24.5) -> (-184.6, 24.3) centre (-184.6, 24.5) ccw
  line L432 (-184.8, 24.5) -> (-184.8, 25.65)
  line L433 (-184.8, 25.65) -> (-185.7, 25.65)
  line L434 (-185.7, 25.65) -> (-185.7, 24.5)
  arc A166 (-185.9, 24.3) -> (-185.7, 24.5) centre (-185.9, 24.5) ccw
  line L435 (-185.9, 24.3) -> (-187.15, 24.3)
  line L436 (-187.15, 24.3) -> (-187.15, 23.2)
  line L437 (-187.15, 23.2) -> (-185.9, 23.2)
  arc A167 (-185.7, 23) -> (-185.9, 23.2) centre (-185.9, 23) ccw
  line L438 (-166.7, 23) -> (-166.7, 21.85)
  line L439 (-166.7, 21.85) -> (-165.8, 21.85)
  line L440 (-165.8, 21.85) -> (-165.8, 23)
  arc A168 (-165.6, 23.2) -> (-165.8, 23) centre (-165.6, 23) ccw
  line L441 (-165.6, 23.2) -> (-164.35, 23.2)
  line L442 (-164.35, 23.2) -> (-164.35, 24.3)
  line L443 (-164.35, 24.3) -> (-165.6, 24.3)
  arc A169 (-165.8, 24.5) -> (-165.6, 24.3) centre (-165.6, 24.5) ccw
  line L444 (-165.8, 24.5) -> (-165.8, 25.65)
  line L445 (-165.8, 25.65) -> (-166.7, 25.65)
  line L446 (-166.7, 25.65) -> (-166.7, 24.5)
  arc A170 (-166.9, 24.3) -> (-166.7, 24.5) centre (-166.9, 24.5) ccw
  line L447 (-166.9, 24.3) -> (-168.15, 24.3)
  line L448 (-168.15, 24.3) -> (-168.15, 23.2)
  line L449 (-168.15, 23.2) -> (-166.9, 23.2)
  arc A171 (-166.7, 23) -> (-166.9, 23.2) centre (-166.9, 23) ccw
  line L450 (-147.7, 23) -> (-147.7, 21.85)
  line L451 (-147.7, 21.85) -> (-146.8, 21.85)
  line L452 (-146.8, 21.85) -> (-146.8, 23)
  arc A172 (-146.6, 23.2) -> (-146.8, 23) centre (-146.6, 23) ccw
  line L453 (-146.6, 23.2) -> (-145.35, 23.2)
  line L454 (-145.35, 23.2) -> (-145.35, 24.3)
  line L455 (-145.35, 24.3) -> (-146.6, 24.3)
  arc A173 (-146.8, 24.5) -> (-146.6, 24.3) centre (-146.6, 24.5) ccw
  line L456 (-146.8, 24.5) -> (-146.8, 25.65)
  line L457 (-146.8, 25.65) -> (-147.7, 25.65)
  line L458 (-147.7, 25.65) -> (-147.7, 24.5)
  arc A174 (-147.9, 24.3) -> (-147.7, 24.5) centre (-147.9, 24.5) ccw
  line L459 (-147.9, 24.3) -> (-149.15, 24.3)
  line L460 (-149.15, 24.3) -> (-149.15, 23.2)
  line L461 (-149.15, 23.2) -> (-147.9, 23.2)
  arc A175 (-147.7, 23) -> (-147.9, 23.2) centre (-147.9, 23) ccw
  line L462 (-204.7, 4) -> (-204.7, 2.85)
  line L463 (-204.7, 2.85) -> (-203.8, 2.85)
  line L464 (-203.8, 2.85) -> (-203.8, 4)
  arc A176 (-203.6, 4.2) -> (-203.8, 4) centre (-203.6, 4) ccw
  line L465 (-203.6, 4.2) -> (-202.35, 4.2)
  line L466 (-202.35, 4.2) -> (-202.35, 5.3)
  line L467 (-202.35, 5.3) -> (-203.6, 5.3)
  arc A177 (-203.8, 5.5) -> (-203.6, 5.3) centre (-203.6, 5.5) ccw
  line L468 (-203.8, 5.5) -> (-203.8, 6.65)
  line L469 (-203.8, 6.65) -> (-204.7, 6.65)
  line L470 (-204.7, 6.65) -> (-204.7, 5.5)
  arc A178 (-204.9, 5.3) -> (-204.7, 5.5) centre (-204.9, 5.5) ccw
  line L471 (-204.9, 5.3) -> (-206.15, 5.3)
  line L472 (-206.15, 5.3) -> (-206.15, 4.2)
  line L473 (-206.15, 4.2) -> (-204.9, 4.2)
  arc A179 (-204.7, 4) -> (-204.9, 4.2) centre (-204.9, 4) ccw
  line L474 (-185.7, 4) -> (-185.7, 2.85)
  line L475 (-185.7, 2.85) -> (-184.8, 2.85)
  line L476 (-184.8, 2.85) -> (-184.8, 4)
  arc A180 (-184.6, 4.2) -> (-184.8, 4) centre (-184.6, 4) ccw
  line L477 (-184.6, 4.2) -> (-183.35, 4.2)
  line L478 (-183.35, 4.2) -> (-183.35, 5.3)
  line L479 (-183.35, 5.3) -> (-184.6, 5.3)
  arc A181 (-184.8, 5.5) -> (-184.6, 5.3) centre (-184.6, 5.5) ccw
  line L480 (-184.8, 5.5) -> (-184.8, 6.65)
  line L481 (-184.8, 6.65) -> (-185.7, 6.65)
  line L482 (-185.7, 6.65) -> (-185.7, 5.5)
  arc A182 (-185.9, 5.3) -> (-185.7, 5.5) centre (-185.9, 5.5) ccw
  line L483 (-185.9, 5.3) -> (-187.15, 5.3)
  line L484 (-187.15, 5.3) -> (-187.15, 4.2)
  line L485 (-187.15, 4.2) -> (-185.9, 4.2)
  arc A183 (-185.7, 4) -> (-185.9, 4.2) centre (-185.9, 4) ccw
  line L486 (-166.7, 4) -> (-166.7, 2.85)
  line L487 (-166.7, 2.85) -> (-165.8, 2.85)
  line L488 (-165.8, 2.85) -> (-165.8, 4)
  arc A184 (-165.6, 4.2) -> (-165.8, 4) centre (-165.6, 4) ccw
  line L489 (-165.6, 4.2) -> (-164.35, 4.2)
  line L490 (-164.35, 4.2) -> (-164.35, 5.3)
  line L491 (-164.35, 5.3) -> (-165.6, 5.3)
  arc A185 (-165.8, 5.5) -> (-165.6, 5.3) centre (-165.6, 5.5) ccw
  line L492 (-165.8, 5.5) -> (-165.8, 6.65)
  line L493 (-165.8, 6.65) -> (-166.7, 6.65)
  line L494 (-166.7, 6.65) -> (-166.7, 5.5)
  arc A186 (-166.9, 5.3) -> (-166.7, 5.5) centre (-166.9, 5.5) ccw
  line L495 (-166.9, 5.3) -> (-168.15, 5.3)
  line L496 (-168.15, 5.3) -> (-168.15, 4.2)
  line L497 (-168.15, 4.2) -> (-166.9, 4.2)
  arc A187 (-166.7, 4) -> (-166.9, 4.2) centre (-166.9, 4) ccw
  line L498 (-147.7, -5.5) -> (-147.7, -6.65)
  line L499 (-147.7, -6.65) -> (-146.8, -6.65)
  line L500 (-146.8, -6.65) -> (-146.8, -5.5)
  arc A188 (-146.6, -5.3) -> (-146.8, -5.5) centre (-146.6, -5.5) ccw
  line L501 (-146.6, -5.3) -> (-145.35, -5.3)
  line L502 (-145.35, -5.3) -> (-145.35, -4.2)
  line L503 (-145.35, -4.2) -> (-146.6, -4.2)
  arc A189 (-146.8, -4) -> (-146.6, -4.2) centre (-146.6, -4) ccw
  line L504 (-146.8, -4) -> (-146.8, -2.85)
  line L505 (-146.8, -2.85) -> (-147.7, -2.85)
  line L506 (-147.7, -2.85) -> (-147.7, -4)
  arc A190 (-147.9, -4.2) -> (-147.7, -4) centre (-147.9, -4) ccw
  line L507 (-147.9, -4.2) -> (-149.15, -4.2)
  line L508 (-149.15, -4.2) -> (-149.15, -5.3)
  line L509 (-149.15, -5.3) -> (-147.9, -5.3)
  arc A191 (-147.7, -5.5) -> (-147.9, -5.3) centre (-147.9, -5.5) ccw
  line L510 (-204.7, -53) -> (-204.7, -54.15)
  line L511 (-204.7, -54.15) -> (-203.8, -54.15)
  line L512 (-203.8, -54.15) -> (-203.8, -53)
  arc A192 (-203.6, -52.8) -> (-203.8, -53) centre (-203.6, -53) ccw
  line L513 (-203.6, -52.8) -> (-202.35, -52.8)
  line L514 (-202.35, -52.8) -> (-202.35, -51.7)
  line L515 (-202.35, -51.7) -> (-203.6, -51.7)
  arc A193 (-203.8, -51.5) -> (-203.6, -51.7) centre (-203.6, -51.5) ccw
  line L516 (-203.8, -51.5) -> (-203.8, -50.35)
  line L517 (-203.8, -50.35) -> (-204.7, -50.35)
  line L518 (-204.7, -50.35) -> (-204.7, -51.5)
  arc A194 (-204.9, -51.7) -> (-204.7, -51.5) centre (-204.9, -51.5) ccw
  line L519 (-204.9, -51.7) -> (-206.15, -51.7)
  line L520 (-206.15, -51.7) -> (-206.15, -52.8)
  line L521 (-206.15, -52.8) -> (-204.9, -52.8)
  arc A195 (-204.7, -53) -> (-204.9, -52.8) centre (-204.9, -53) ccw
  line L522 (-185.7, -53) -> (-185.7, -54.15)
  line L523 (-185.7, -54.15) -> (-184.8, -54.15)
  line L524 (-184.8, -54.15) -> (-184.8, -53)
  arc A196 (-184.6, -52.8) -> (-184.8, -53) centre (-184.6, -53) ccw
  line L525 (-184.6, -52.8) -> (-183.35, -52.8)
  line L526 (-183.35, -52.8) -> (-183.35, -51.7)
  line L527 (-183.35, -51.7) -> (-184.6, -51.7)
  arc A197 (-184.8, -51.5) -> (-184.6, -51.7) centre (-184.6, -51.5) ccw
  line L528 (-184.8, -51.5) -> (-184.8, -50.35)
  line L529 (-184.8, -50.35) -> (-185.7, -50.35)
  line L530 (-185.7, -50.35) -> (-185.7, -51.5)
  arc A198 (-185.9, -51.7) -> (-185.7, -51.5) centre (-185.9, -51.5) ccw
  line L531 (-185.9, -51.7) -> (-187.15, -51.7)
  line L532 (-187.15, -51.7) -> (-187.15, -52.8)
  line L533 (-187.15, -52.8) -> (-185.9, -52.8)
  arc A199 (-185.7, -53) -> (-185.9, -52.8) centre (-185.9, -53) ccw
  line L534 (-166.7, -53) -> (-166.7, -54.15)
  line L535 (-166.7, -54.15) -> (-165.8, -54.15)
  line L536 (-165.8, -54.15) -> (-165.8, -53)
  arc A200 (-165.6, -52.8) -> (-165.8, -53) centre (-165.6, -53) ccw
  line L537 (-165.6, -52.8) -> (-164.35, -52.8)
  line L538 (-164.35, -52.8) -> (-164.35, -51.7)
  line L539 (-164.35, -51.7) -> (-165.6, -51.7)
  arc A201 (-165.8, -51.5) -> (-165.6, -51.7) centre (-165.6, -51.5) ccw
  line L540 (-165.8, -51.5) -> (-165.8, -50.35)
  line L541 (-165.8, -50.35) -> (-166.7, -50.35)
  line L542 (-166.7, -50.35) -> (-166.7, -51.5)
  arc A202 (-166.9, -51.7) -> (-166.7, -51.5) centre (-166.9, -51.5) ccw
  line L543 (-166.9, -51.7) -> (-168.15, -51.7)
  line L544 (-168.15, -51.7) -> (-168.15, -52.8)
  line L545 (-168.15, -52.8) -> (-166.9, -52.8)
  arc A203 (-166.7, -53) -> (-166.9, -52.8) centre (-166.9, -53) ccw
  line L546 (-147.7, -43.5) -> (-147.7, -44.65)
  line L547 (-147.7, -44.65) -> (-146.8, -44.65)
  line L548 (-146.8, -44.65) -> (-146.8, -43.5)
  arc A204 (-146.6, -43.3) -> (-146.8, -43.5) centre (-146.6, -43.5) ccw
  line L549 (-146.6, -43.3) -> (-145.35, -43.3)
  line L550 (-145.35, -43.3) -> (-145.35, -42.2)
  line L551 (-145.35, -42.2) -> (-146.6, -42.2)
  arc A205 (-146.8, -42) -> (-146.6, -42.2) centre (-146.6, -42) ccw
  line L552 (-146.8, -42) -> (-146.8, -40.85)
  line L553 (-146.8, -40.85) -> (-147.7, -40.85)
  line L554 (-147.7, -40.85) -> (-147.7, -42)
  arc A206 (-147.9, -42.2) -> (-147.7, -42) centre (-147.9, -42) ccw
  line L555 (-147.9, -42.2) -> (-149.15, -42.2)
  line L556 (-149.15, -42.2) -> (-149.15, -43.3)
  line L557 (-149.15, -43.3) -> (-147.9, -43.3)
  arc A207 (-147.7, -43.5) -> (-147.9, -43.3) centre (-147.9, -43.5) ccw
  line L558 (-166.7, -34) -> (-166.7, -35.15)
  line L559 (-166.7, -35.15) -> (-165.8, -35.15)
  line L560 (-165.8, -35.15) -> (-165.8, -34)
  arc A208 (-165.6, -33.8) -> (-165.8, -34) centre (-165.6, -34) ccw
  line L561 (-165.6, -33.8) -> (-164.35, -33.8)
  line L562 (-164.35, -33.8) -> (-164.35, -32.7)
  line L563 (-164.35, -32.7) -> (-165.6, -32.7)
  arc A209 (-165.8, -32.5) -> (-165.6, -32.7) centre (-165.6, -32.5) ccw
  line L564 (-165.8, -32.5) -> (-165.8, -31.35)
  line L565 (-165.8, -31.35) -> (-166.7, -31.35)
  line L566 (-166.7, -31.35) -> (-166.7, -32.5)
  arc A210 (-166.9, -32.7) -> (-166.7, -32.5) centre (-166.9, -32.5) ccw
  line L567 (-166.9, -32.7) -> (-168.15, -32.7)
  line L568 (-168.15, -32.7) -> (-168.15, -33.8)
  line L569 (-168.15, -33.8) -> (-166.9, -33.8)
  arc A211 (-166.7, -34) -> (-166.9, -33.8) centre (-166.9, -34) ccw
  line L570 (-185.7, -34) -> (-185.7, -35.15)
  line L571 (-185.7, -35.15) -> (-184.8, -35.15)
  line L572 (-184.8, -35.15) -> (-184.8, -34)
  arc A212 (-184.6, -33.8) -> (-184.8, -34) centre (-184.6, -34) ccw
  line L573 (-184.6, -33.8) -> (-183.35, -33.8)
  line L574 (-183.35, -33.8) -> (-183.35, -32.7)
  line L575 (-183.35, -32.7) -> (-184.6, -32.7)
  arc A213 (-184.8, -32.5) -> (-184.6, -32.7) centre (-184.6, -32.5) ccw
  line L576 (-184.8, -32.5) -> (-184.8, -31.35)
  line L577 (-184.8, -31.35) -> (-185.7, -31.35)
  line L578 (-185.7, -31.35) -> (-185.7, -32.5)
  arc A214 (-185.9, -32.7) -> (-185.7, -32.5) centre (-185.9, -32.5) ccw
  line L579 (-185.9, -32.7) -> (-187.15, -32.7)
  line L580 (-187.15, -32.7) -> (-187.15, -33.8)
  line L581 (-187.15, -33.8) -> (-185.9, -33.8)
  arc A215 (-185.7, -34) -> (-185.9, -33.8) centre (-185.9, -34) ccw
  line L582 (-204.7, -34) -> (-204.7, -35.15)
  line L583 (-204.7, -35.15) -> (-203.8, -35.15)
  line L584 (-203.8, -35.15) -> (-203.8, -34)
  arc A216 (-203.6, -33.8) -> (-203.8, -34) centre (-203.6, -34) ccw
  line L585 (-203.6, -33.8) -> (-202.35, -33.8)
  line L586 (-202.35, -33.8) -> (-202.35, -32.7)
  line L587 (-202.35, -32.7) -> (-203.6, -32.7)
  arc A217 (-203.8, -32.5) -> (-203.6, -32.7) centre (-203.6, -32.5) ccw
  line L588 (-203.8, -32.5) -> (-203.8, -31.35)
  line L589 (-203.8, -31.35) -> (-204.7, -31.35)
  line L590 (-204.7, -31.35) -> (-204.7, -32.5)
  arc A218 (-204.9, -32.7) -> (-204.7, -32.5) centre (-204.9, -32.5) ccw
  line L591 (-204.9, -32.7) -> (-206.15, -32.7)
  line L592 (-206.15, -32.7) -> (-206.15, -33.8)
  line L593 (-206.15, -33.8) -> (-204.9, -33.8)
  arc A219 (-204.7, -34) -> (-204.9, -33.8) centre (-204.9, -34) ccw
  line L594 (-204.7, -15) -> (-204.7, -16.15)
  line L595 (-204.7, -16.15) -> (-203.8, -16.15)
  line L596 (-203.8, -16.15) -> (-203.8, -15)
  arc A220 (-203.6, -14.8) -> (-203.8, -15) centre (-203.6, -15) ccw
  line L597 (-203.6, -14.8) -> (-202.35, -14.8)
  line L598 (-202.35, -14.8) -> (-202.35, -13.7)
  line L599 (-202.35, -13.7) -> (-203.6, -13.7)
  arc A221 (-203.8, -13.5) -> (-203.6, -13.7) centre (-203.6, -13.5) ccw
  line L600 (-203.8, -13.5) -> (-203.8, -12.35)
  line L601 (-203.8, -12.35) -> (-204.7, -12.35)
  line L602 (-204.7, -12.35) -> (-204.7, -13.5)
  arc A222 (-204.9, -13.7) -> (-204.7, -13.5) centre (-204.9, -13.5) ccw
  line L603 (-204.9, -13.7) -> (-206.15, -13.7)
  line L604 (-206.15, -13.7) -> (-206.15, -14.8)
  line L605 (-206.15, -14.8) -> (-204.9, -14.8)
  arc A223 (-204.7, -15) -> (-204.9, -14.8) centre (-204.9, -15) ccw
  line L606 (-185.7, -15) -> (-185.7, -16.15)
  line L607 (-185.7, -16.15) -> (-184.8, -16.15)
  line L608 (-184.8, -16.15) -> (-184.8, -15)
  arc A224 (-184.6, -14.8) -> (-184.8, -15) centre (-184.6, -15) ccw
  line L609 (-184.6, -14.8) -> (-183.35, -14.8)
  line L610 (-183.35, -14.8) -> (-183.35, -13.7)
  line L611 (-183.35, -13.7) -> (-184.6, -13.7)
  arc A225 (-184.8, -13.5) -> (-184.6, -13.7) centre (-184.6, -13.5) ccw
  line L612 (-184.8, -13.5) -> (-184.8, -12.35)
  line L613 (-184.8, -12.35) -> (-185.7, -12.35)
  line L614 (-185.7, -12.35) -> (-185.7, -13.5)
  arc A226 (-185.9, -13.7) -> (-185.7, -13.5) centre (-185.9, -13.5) ccw
  line L615 (-185.9, -13.7) -> (-187.15, -13.7)
  line L616 (-187.15, -13.7) -> (-187.15, -14.8)
  line L617 (-187.15, -14.8) -> (-185.9, -14.8)
  arc A227 (-185.7, -15) -> (-185.9, -14.8) centre (-185.9, -15) ccw
  line L618 (-166.7, -15) -> (-166.7, -16.15)
  line L619 (-166.7, -16.15) -> (-165.8, -16.15)
  line L620 (-165.8, -16.15) -> (-165.8, -15)
  arc A228 (-165.6, -14.8) -> (-165.8, -15) centre (-165.6, -15) ccw
  line L621 (-165.6, -14.8) -> (-164.35, -14.8)
  line L622 (-164.35, -14.8) -> (-164.35, -13.7)
  line L623 (-164.35, -13.7) -> (-165.6, -13.7)
  arc A229 (-165.8, -13.5) -> (-165.6, -13.7) centre (-165.6, -13.5) ccw
  line L624 (-165.8, -13.5) -> (-165.8, -12.35)
  line L625 (-165.8, -12.35) -> (-166.7, -12.35)
  line L626 (-166.7, -12.35) -> (-166.7, -13.5)
  arc A230 (-166.9, -13.7) -> (-166.7, -13.5) centre (-166.9, -13.5) ccw
  line L627 (-166.9, -13.7) -> (-168.15, -13.7)
  line L628 (-168.15, -13.7) -> (-168.15, -14.8)
  line L629 (-168.15, -14.8) -> (-166.9, -14.8)
  arc A231 (-166.7, -15) -> (-166.9, -14.8) centre (-166.9, -15) ccw
  line L630 (-123.95, -53) -> (-123.95, -54.15)
  line L631 (-123.95, -54.15) -> (-123.05, -54.15)
  line L632 (-123.05, -54.15) -> (-123.05, -53)
  arc A232 (-122.85, -52.8) -> (-123.05, -53) centre (-122.85, -53) ccw
  line L633 (-122.85, -52.8) -> (-121.6, -52.8)
  line L634 (-121.6, -52.8) -> (-121.6, -51.7)
  line L635 (-121.6, -51.7) -> (-122.85, -51.7)
  arc A233 (-123.05, -51.5) -> (-122.85, -51.7) centre (-122.85, -51.5) ccw
  line L636 (-123.05, -51.5) -> (-123.05, -50.35)
  line L637 (-123.05, -50.35) -> (-123.95, -50.35)
  line L638 (-123.95, -50.35) -> (-123.95, -51.5)
  arc A234 (-124.15, -51.7) -> (-123.95, -51.5) centre (-124.15, -51.5) ccw
  line L639 (-124.15, -51.7) -> (-125.4, -51.7)
  line L640 (-125.4, -51.7) -> (-125.4, -52.8)
  line L641 (-125.4, -52.8) -> (-124.15, -52.8)
  arc A235 (-123.95, -53) -> (-124.15, -52.8) centre (-124.15, -53) ccw
  line L642 (-104.95, -53) -> (-104.95, -54.15)
  line L643 (-104.95, -54.15) -> (-104.05, -54.15)
  line L644 (-104.05, -54.15) -> (-104.05, -53)
  arc A236 (-103.85, -52.8) -> (-104.05, -53) centre (-103.85, -53) ccw
  line L645 (-103.85, -52.8) -> (-102.6, -52.8)
  line L646 (-102.6, -52.8) -> (-102.6, -51.7)
  line L647 (-102.6, -51.7) -> (-103.85, -51.7)
  arc A237 (-104.05, -51.5) -> (-103.85, -51.7) centre (-103.85, -51.5) ccw
  line L648 (-104.05, -51.5) -> (-104.05, -50.35)
  line L649 (-104.05, -50.35) -> (-104.95, -50.35)
  line L650 (-104.95, -50.35) -> (-104.95, -51.5)
  arc A238 (-105.15, -51.7) -> (-104.95, -51.5) centre (-105.15, -51.5) ccw
  line L651 (-105.15, -51.7) -> (-106.4, -51.7)
  line L652 (-106.4, -51.7) -> (-106.4, -52.8)
  line L653 (-106.4, -52.8) -> (-105.15, -52.8)
  arc A239 (-104.95, -53) -> (-105.15, -52.8) centre (-105.15, -53) ccw
  line L654 (-104.95, -34) -> (-104.95, -35.15)
  line L655 (-104.95, -35.15) -> (-104.05, -35.15)
  line L656 (-104.05, -35.15) -> (-104.05, -34)
  arc A240 (-103.85, -33.8) -> (-104.05, -34) centre (-103.85, -34) ccw
  line L657 (-103.85, -33.8) -> (-102.6, -33.8)
  line L658 (-102.6, -33.8) -> (-102.6, -32.7)
  line L659 (-102.6, -32.7) -> (-103.85, -32.7)
  arc A241 (-104.05, -32.5) -> (-103.85, -32.7) centre (-103.85, -32.5) ccw
  line L660 (-104.05, -32.5) -> (-104.05, -31.35)
  line L661 (-104.05, -31.35) -> (-104.95, -31.35)
  line L662 (-104.95, -31.35) -> (-104.95, -32.5)
  arc A242 (-105.15, -32.7) -> (-104.95, -32.5) centre (-105.15, -32.5) ccw
  line L663 (-105.15, -32.7) -> (-106.4, -32.7)
  line L664 (-106.4, -32.7) -> (-106.4, -33.8)
  line L665 (-106.4, -33.8) -> (-105.15, -33.8)
  arc A243 (-104.95, -34) -> (-105.15, -33.8) centre (-105.15, -34) ccw
  line L666 (-85.95, -53) -> (-85.95, -54.15)
  line L667 (-85.95, -54.15) -> (-85.05, -54.15)
  line L668 (-85.05, -54.15) -> (-85.05, -53)
  arc A244 (-84.85, -52.8) -> (-85.05, -53) centre (-84.85, -53) ccw
  line L669 (-84.85, -52.8) -> (-83.6, -52.8)
  line L670 (-83.6, -52.8) -> (-83.6, -51.7)
  line L671 (-83.6, -51.7) -> (-84.85, -51.7)
  arc A245 (-85.05, -51.5) -> (-84.85, -51.7) centre (-84.85, -51.5) ccw
  line L672 (-85.05, -51.5) -> (-85.05, -50.35)
  line L673 (-85.05, -50.35) -> (-85.95, -50.35)
  line L674 (-85.95, -50.35) -> (-85.95, -51.5)
  arc A246 (-86.15, -51.7) -> (-85.95, -51.5) centre (-86.15, -51.5) ccw
  line L675 (-86.15, -51.7) -> (-87.4, -51.7)
  line L676 (-87.4, -51.7) -> (-87.4, -52.8)
  line L677 (-87.4, -52.8) -> (-86.15, -52.8)
  arc A247 (-85.95, -53) -> (-86.15, -52.8) centre (-86.15, -53) ccw
  line L678 (-59.825, -53) -> (-59.825, -54.15)
  line L679 (-59.825, -54.15) -> (-58.925, -54.15)
  line L680 (-58.925, -54.15) -> (-58.925, -53)
  arc A248 (-58.725, -52.8) -> (-58.925, -53) centre (-58.725, -53) ccw
  line L681 (-58.725, -52.8) -> (-57.475, -52.8)
  line L682 (-57.475, -52.8) -> (-57.475, -51.7)
  line L683 (-57.475, -51.7) -> (-58.725, -51.7)
  arc A249 (-58.925, -51.5) -> (-58.725, -51.7) centre (-58.725, -51.5) ccw
  line L684 (-58.925, -51.5) -> (-58.925, -50.35)
  line L685 (-58.925, -50.35) -> (-59.825, -50.35)
  line L686 (-59.825, -50.35) -> (-59.825, -51.5)
  arc A250 (-60.025, -51.7) -> (-59.825, -51.5) centre (-60.025, -51.5) ccw
  line L687 (-60.025, -51.7) -> (-61.275, -51.7)
  line L688 (-61.275, -51.7) -> (-61.275, -52.8)
  line L689 (-61.275, -52.8) -> (-60.025, -52.8)
  arc A251 (-59.825, -53) -> (-60.025, -52.8) centre (-60.025, -53) ccw
  line L690 (-57.45, 4) -> (-57.45, 2.85)
  line L691 (-57.45, 2.85) -> (-56.55, 2.85)
  line L692 (-56.55, 2.85) -> (-56.55, 4)
  arc A252 (-56.35, 4.2) -> (-56.55, 4) centre (-56.35, 4) ccw
  line L693 (-56.35, 4.2) -> (-55.1, 4.2)
  line L694 (-55.1, 4.2) -> (-55.1, 5.3)
  line L695 (-55.1, 5.3) -> (-56.35, 5.3)
  arc A253 (-56.55, 5.5) -> (-56.35, 5.3) centre (-56.35, 5.5) ccw
  line L696 (-56.55, 5.5) -> (-56.55, 6.65)
  line L697 (-56.55, 6.65) -> (-57.45, 6.65)
  line L698 (-57.45, 6.65) -> (-57.45, 5.5)
  arc A254 (-57.65, 5.3) -> (-57.45, 5.5) centre (-57.65, 5.5) ccw
  line L699 (-57.65, 5.3) -> (-58.9, 5.3)
  line L700 (-58.9, 5.3) -> (-58.9, 4.2)
  line L701 (-58.9, 4.2) -> (-57.65, 4.2)
  arc A255 (-57.45, 4) -> (-57.65, 4.2) centre (-57.65, 4) ccw
  line L702 (-55.075, -15) -> (-55.075, -16.15)
  line L703 (-55.075, -16.15) -> (-54.175, -16.15)
  line L704 (-54.175, -16.15) -> (-54.175, -15)
  arc A256 (-53.975, -14.8) -> (-54.175, -15) centre (-53.975, -15) ccw
  line L705 (-53.975, -14.8) -> (-52.725, -14.8)
  line L706 (-52.725, -14.8) -> (-52.725, -13.7)
  line L707 (-52.725, -13.7) -> (-53.975, -13.7)
  arc A257 (-54.175, -13.5) -> (-53.975, -13.7) centre (-53.975, -13.5) ccw
  line L708 (-54.175, -13.5) -> (-54.175, -12.35)
  line L709 (-54.175, -12.35) -> (-55.075, -12.35)
  line L710 (-55.075, -12.35) -> (-55.075, -13.5)
  arc A258 (-55.275, -13.7) -> (-55.075, -13.5) centre (-55.275, -13.5) ccw
  line L711 (-55.275, -13.7) -> (-56.525, -13.7)
  line L712 (-56.525, -13.7) -> (-56.525, -14.8)
  line L713 (-56.525, -14.8) -> (-55.275, -14.8)
  arc A259 (-55.075, -15) -> (-55.275, -14.8) centre (-55.275, -15) ccw
  line L714 (-50.325, -34) -> (-50.325, -35.15)
  line L715 (-50.325, -35.15) -> (-49.425, -35.15)
  line L716 (-49.425, -35.15) -> (-49.425, -34)
  arc A260 (-49.225, -33.8) -> (-49.425, -34) centre (-49.225, -34) ccw